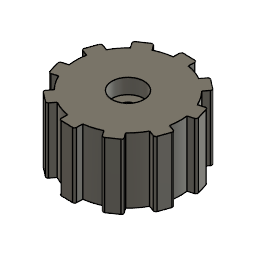
Tank tread gear (Autodesk Fusion 360 design; units mm, degrees)
part number: 2026-08-01-11-00-48-314
Autodesk Fusion 360 part; units mm, degrees
sketch "Sketch1" plane through (0, 0, 0) normal (0, 1, 0) x (1, 0, 0)
  circle A0 centre (0, 0) radius 8
  line L0 (1.3935, 7.8777) -> (1.4168, 8.8274)
  line L1 (1.1242, 9.1347) -> (-0.6752, 9.1788)
  line L2 (-0.9825, 8.8862) -> (-1.0058, 7.9365)
  line L3 (-3.503, 7.1923) -> (-4.0424, 7.9743)
  line L4 (-4.4597, 8.0509) -> (-5.9414, 7.0289)
  line L5 (-6.018, 6.6116) -> (-5.4786, 5.8296)
  line L6 (-7.0615, 3.7597) -> (-7.9575, 4.0753)
  line L7 (-8.3402, 3.892) -> (-8.9382, 2.1942)
  line L8 (-8.7549, 1.8116) -> (-7.8589, 1.496)
  line L9 (-7.9228, -1.109) -> (-8.8332, -1.3804)
  line L10 (-9.035, -1.7535) -> (-8.5209, -3.4786)
  line L11 (-8.1477, -3.6804) -> (-7.2373, -3.4091)
  line L12 (-5.7578, -5.5541) -> (-6.3348, -6.3087)
  line L13 (-6.2788, -6.7293) -> (-4.8489, -7.8227)
  line L14 (-4.4284, -7.7666) -> (-3.8513, -7.012)
  line L15 (-1.3935, -7.8777) -> (-1.4168, -8.8274)
  line L16 (-1.1242, -9.1347) -> (0.6752, -9.1788)
  line L17 (0.9825, -8.8862) -> (1.0058, -7.9365)
  line L18 (3.503, -7.1923) -> (4.0424, -7.9743)
  line L19 (4.4597, -8.0509) -> (5.9414, -7.0289)
  line L20 (6.018, -6.6116) -> (5.4786, -5.8296)
  line L21 (7.0615, -3.7597) -> (7.9575, -4.0753)
  line L22 (8.3402, -3.892) -> (8.9382, -2.1942)
  line L23 (8.7549, -1.8116) -> (7.8589, -1.496)
  line L24 (7.9228, 1.109) -> (8.8332, 1.3804)
  line L25 (9.035, 1.7535) -> (8.5209, 3.4786)
  line L26 (8.1477, 3.6804) -> (7.2373, 3.4091)
  line L27 (5.7578, 5.5541) -> (6.3348, 6.3087)
  line L28 (6.2788, 6.7293) -> (4.8489, 7.8227)
  line L29 (4.4284, 7.7666) -> (3.8513, 7.012)
  arc A1 (-0.6752, 9.1788) -> (-0.9825, 8.8862) centre (-0.6826, 8.8789) ccw
  arc A2 (1.4168, 8.8274) -> (1.1242, 9.1347) centre (1.1169, 8.8348) ccw
  arc A3 (4.8489, 7.8227) -> (4.4284, 7.7666) centre (4.6667, 7.5844) ccw
  arc A4 (6.3348, 6.3087) -> (6.2788, 6.7293) centre (6.0965, 6.491) ccw
  arc A5 (8.5209, 3.4786) -> (8.1477, 3.6804) centre (8.2334, 3.3929) ccw
  arc A6 (8.8332, 1.3804) -> (9.035, 1.7535) centre (8.7475, 1.6679) ccw
  arc A7 (8.9382, -2.1942) -> (8.7549, -1.8116) centre (8.6552, -2.0946) ccw
  arc A8 (7.9575, -4.0753) -> (8.3402, -3.892) centre (8.0572, -3.7923) ccw
  arc A9 (5.9414, -7.0289) -> (6.018, -6.6116) centre (5.7711, -6.782) ccw
  arc A10 (4.0424, -7.9743) -> (4.4597, -8.0509) centre (4.2894, -7.804) ccw
  arc A11 (0.6752, -9.1788) -> (0.9825, -8.8862) centre (0.6826, -8.8789) ccw
  arc A12 (-1.4168, -8.8274) -> (-1.1242, -9.1347) centre (-1.1169, -8.8348) ccw
  arc A13 (-4.8489, -7.8227) -> (-4.4284, -7.7666) centre (-4.6667, -7.5844) ccw
  arc A14 (-6.3348, -6.3087) -> (-6.2788, -6.7293) centre (-6.0965, -6.491) ccw
  arc A15 (-8.5209, -3.4786) -> (-8.1477, -3.6804) centre (-8.2334, -3.3929) ccw
  arc A16 (-8.8332, -1.3804) -> (-9.035, -1.7535) centre (-8.7475, -1.6679) ccw
  arc A17 (-7.9575, 4.0753) -> (-8.3402, 3.892) centre (-8.0572, 3.7923) ccw
  arc A18 (-8.9382, 2.1942) -> (-8.7549, 1.8116) centre (-8.6552, 2.0946) ccw
  arc A19 (-4.0424, 7.9743) -> (-4.4597, 8.0509) centre (-4.2894, 7.804) ccw
  arc A20 (-5.9414, 7.0289) -> (-6.018, 6.6116) centre (-5.7711, 6.782) ccw
  point P0 (-0.9751, 9.1862)
  dimension "d1" = 16
  dimension "d2" = 2.4
  dimension "d3" = 1.25
  dimension "d6" = 0.3
  constraint coincident A0.centre origin
  constraint coincident A0 L2.end
  constraint coincident A0 L0.start
  constraint parallel L0 L2
  constraint perpendicular L1 L2
  constraint coincident P0 L1
  constraint coincident P0 L2
  constraint tangent L1 A1
  constraint tangent L2 A1
  constraint tangent L0 A2
  constraint tangent L1 A2
  constraint equal A1 A2
  constraint tangent L28 A3
  constraint tangent L29 A3
  constraint equal A1 A3
  constraint tangent L27 A4
  constraint tangent L28 A4
  constraint equal A1 A4
  constraint tangent L25 A5
  constraint tangent L26 A5
  constraint equal A1 A5
  constraint tangent L24 A6
  constraint tangent L25 A6
  constraint equal A1 A6
  constraint tangent L22 A7
  constraint tangent L23 A7
  constraint equal A1 A7
  constraint tangent L21 A8
  constraint tangent L22 A8
  constraint equal A1 A8
  constraint tangent L19 A9
  constraint tangent L20 A9
  constraint equal A1 A9
  constraint tangent L18 A10
  constraint tangent L19 A10
  constraint equal A1 A10
  constraint tangent L16 A11
  constraint tangent L17 A11
  constraint equal A1 A11
  constraint tangent L15 A12
  constraint tangent L16 A12
  constraint equal A1 A12
  constraint tangent L13 A13
  constraint tangent L14 A13
  constraint equal A1 A13
  constraint tangent L12 A14
  constraint tangent L13 A14
  constraint equal A1 A14
  constraint tangent L10 A15
  constraint tangent L11 A15
  constraint equal A1 A15
  constraint tangent L9 A16
  constraint tangent L10 A16
  constraint equal A1 A16
  constraint tangent L6 A17
  constraint tangent L7 A17
  constraint equal A1 A17
  constraint tangent L7 A18
  constraint tangent L8 A18
  constraint equal A1 A18
  constraint tangent L3 A19
  constraint tangent L4 A19
  constraint equal A1 A19
  constraint tangent L4 A20
  constraint tangent L5 A20
  constraint equal A1 A20
  measures "d1" diameter of A0
  measures "d2" distance of L2.end L0.start
  measures "d3" distance of L2.end P0
  measures "d6" radius of A1
extrude "Extrude1" add sketch "Sketch1" along normal blind 10
sketch "Sketch2" plane through (0, 10, 0) normal (0, 1, 0) x (-1, 0, 0)
  arc A0 (5.9414, -7.0289) -> (6.018, -6.6116) centre (5.7711, -6.782) ccw
  line L0 (6.018, -6.6116) -> (5.4786, -5.8296)
  arc A1 (5.4786, -5.8296) -> (7.0615, -3.7597) centre (0, 0) ccw
  line L1 (7.0615, -3.7597) -> (7.9575, -4.0753)
  arc A2 (7.9575, -4.0753) -> (8.3402, -3.892) centre (8.0572, -3.7923) ccw
  line L2 (8.3402, -3.892) -> (8.9382, -2.1942)
  arc A3 (8.9382, -2.1942) -> (8.7549, -1.8116) centre (8.6552, -2.0946) ccw
  line L3 (8.7549, -1.8116) -> (7.8589, -1.496)
  arc A4 (7.8589, -1.496) -> (7.9228, 1.109) centre (0, 0) ccw
  line L4 (7.9228, 1.109) -> (8.8332, 1.3804)
  arc A5 (8.8332, 1.3804) -> (9.035, 1.7535) centre (8.7475, 1.6679) ccw
  line L5 (9.035, 1.7535) -> (8.5209, 3.4786)
  arc A6 (8.5209, 3.4786) -> (8.1477, 3.6804) centre (8.2334, 3.3929) ccw
  line L6 (8.1477, 3.6804) -> (7.2373, 3.4091)
  arc A7 (7.2373, 3.4091) -> (5.7578, 5.5541) centre (0, 0) ccw
  line L7 (5.7578, 5.5541) -> (6.3348, 6.3087)
  arc A8 (6.3348, 6.3087) -> (6.2788, 6.7293) centre (6.0965, 6.491) ccw
  line L8 (6.2788, 6.7293) -> (4.8489, 7.8227)
  arc A9 (4.8489, 7.8227) -> (4.4284, 7.7666) centre (4.6667, 7.5844) ccw
  line L9 (4.4284, 7.7666) -> (3.8513, 7.012)
  arc A10 (3.8513, 7.012) -> (1.3935, 7.8777) centre (0, 0) ccw
  line L10 (1.3935, 7.8777) -> (1.4168, 8.8274)
  arc A11 (1.4168, 8.8274) -> (1.1242, 9.1347) centre (1.1169, 8.8348) ccw
  line L11 (1.1242, 9.1347) -> (-0.6752, 9.1788)
  arc A12 (-0.6752, 9.1788) -> (-0.9825, 8.8862) centre (-0.6826, 8.8789) ccw
  line L12 (-0.9825, 8.8862) -> (-1.0058, 7.9365)
  arc A13 (-1.0058, 7.9365) -> (-3.503, 7.1923) centre (0, 0) ccw
  line L13 (-3.503, 7.1923) -> (-4.0424, 7.9743)
  arc A14 (-4.0424, 7.9743) -> (-4.4597, 8.0509) centre (-4.2894, 7.804) ccw
  line L14 (-4.4597, 8.0509) -> (-5.9414, 7.0289)
  arc A15 (-5.9414, 7.0289) -> (-6.018, 6.6116) centre (-5.7711, 6.782) ccw
  line L15 (-6.018, 6.6116) -> (-5.4786, 5.8296)
  arc A16 (-5.4786, 5.8296) -> (-7.0615, 3.7597) centre (0, 0) ccw
  line L16 (-7.0615, 3.7597) -> (-7.9575, 4.0753)
  arc A17 (-7.9575, 4.0753) -> (-8.3402, 3.892) centre (-8.0572, 3.7923) ccw
  line L17 (-8.3402, 3.892) -> (-8.9382, 2.1942)
  arc A18 (-8.9382, 2.1942) -> (-8.7549, 1.8116) centre (-8.6552, 2.0946) ccw
  line L18 (-8.7549, 1.8116) -> (-7.8589, 1.496)
  arc A19 (-7.8589, 1.496) -> (-7.9228, -1.109) centre (0, 0) ccw
  line L19 (-7.9228, -1.109) -> (-8.8332, -1.3804)
  arc A20 (-8.8332, -1.3804) -> (-9.035, -1.7535) centre (-8.7475, -1.6679) ccw
  line L20 (-9.035, -1.7535) -> (-8.5209, -3.4786)
  arc A21 (-8.5209, -3.4786) -> (-8.1477, -3.6804) centre (-8.2334, -3.3929) ccw
  line L21 (-8.1477, -3.6804) -> (-7.2373, -3.4091)
  arc A22 (-7.2373, -3.4091) -> (-5.7578, -5.5541) centre (0, 0) ccw
  line L22 (-5.7578, -5.5541) -> (-6.3348, -6.3087)
  arc A23 (-6.3348, -6.3087) -> (-6.2788, -6.7293) centre (-6.0965, -6.491) ccw
  line L23 (-6.2788, -6.7293) -> (-4.8489, -7.8227)
  arc A24 (-4.8489, -7.8227) -> (-4.4284, -7.7666) centre (-4.6667, -7.5844) ccw
  line L24 (-4.4284, -7.7666) -> (-3.8513, -7.012)
  arc A25 (-3.8513, -7.012) -> (-1.3935, -7.8777) centre (0, 0) ccw
  line L25 (-1.3935, -7.8777) -> (-1.4168, -8.8274)
  arc A26 (-1.4168, -8.8274) -> (-1.1242, -9.1347) centre (-1.1169, -8.8348) ccw
  line L26 (-1.1242, -9.1347) -> (0.6752, -9.1788)
  arc A27 (0.6752, -9.1788) -> (0.9825, -8.8862) centre (0.6826, -8.8789) ccw
  line L27 (0.9825, -8.8862) -> (1.0058, -7.9365)
  arc A28 (1.0058, -7.9365) -> (3.503, -7.1923) centre (0, 0) ccw
  line L28 (3.503, -7.1923) -> (4.0424, -7.9743)
  arc A29 (4.0424, -7.9743) -> (4.4597, -8.0509) centre (4.2894, -7.804) ccw
  line L29 (4.4597, -8.0509) -> (5.9414, -7.0289)
  circle A30 centre (0, 0) radius 2.45
  dimension "d9" = 4.9
  constraint concentric A1 A30
  measures "d9" diameter of A30
extrude "Extrude2" cut sketch "Sketch2" against normal blind 2.3 contours A30
sketch "Sketch3" plane through (0, 7.7, 0) normal (0, 1, 0) x (-1, 0, 0)
  circle A0 centre (0, 0) radius 2.45
  circle A1 centre (0, 0) radius 1.05
  dimension "d12" = 2.1
  constraint concentric A0 A1
  measures "d12" diameter of A1
extrude "Extrude3" cut sketch "Sketch3" against normal blind 44.519 contours A1
